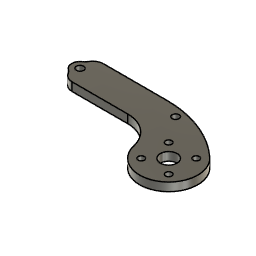
dribbler (Autodesk Fusion 360 archive; units mm, degrees)
design "ドリブラー1-1"
Autodesk Fusion 360 part; units mm, degrees
sketch "スケッチ1" plane through (0, 0, 2.2603) normal (0, 0, -1) x (1, 0, 0)
  circle A0 centre (-0.3584, 25.4794) radius 1.5
  circle A1 centre (12.7938, 12.3272) radius 1.5
  circle A2 centre (6.2177, 18.9033) radius 4
  arc A3 (17.8871, 26.363) -> (13.6774, 30.5727) centre (6.2177, 18.9033) ccw
  arc A4 (-1.242, 30.5727) -> (13.6774, 30.5727) centre (6.2177, 40.3986) ccw
  arc A5 (-1.242, 30.5727) -> (-5.4517, 26.363) centre (6.2177, 18.9033) ccw
  arc A6 (-5.4517, 11.4436) -> (-5.4517, 26.363) centre (-15.2776, 18.9033) ccw
  arc A7 (-5.4517, 11.4436) -> (-1.242, 7.2339) centre (6.2177, 18.9033) ccw
  arc A8 (13.6774, 7.2339) -> (-1.242, 7.2339) centre (6.2177, -2.592) ccw
  arc A9 (13.6774, 7.2339) -> (17.8871, 11.4436) centre (6.2177, 18.9033) ccw
  arc A10 (17.8871, 26.363) -> (17.8871, 11.4436) centre (27.713, 18.9033) ccw
  circle A11 centre (-0.3584, 12.3272) radius 1.5
  circle A12 centre (12.7938, 25.4794) radius 1.5
  circle A13 centre (12.7938, 25.4794) radius 1.6
  circle A14 centre (-0.3584, 12.3272) radius 1.6
  circle A15 centre (12.7938, 12.3272) radius 1.6
  circle A16 centre (-0.3584, 25.4794) radius 1.6
  circle A17 centre (6.2177, 18.9033) radius 13.9
  line L0 (12.7938, 12.3272) -> (-0.3584, 12.3272)
  line L1 (6.2177, 12.3272) -> (6.2177, 10.3272)
  line L2 (6.2177, 10.3272) -> (-53.7823, 10.3272)
  line L3 (6.2177, 18.9033) -> (-0.3584, 12.3272)
  line L4 (-0.3584, 12.3272) -> (-2.3584, 10.3272)
  line L5 (6.2177, 18.9033) -> (-7.6823, 18.9033)
  line L6 (-7.6823, 18.9033) -> (-7.6823, 10.3272)
  line L7 (6.2177, 18.9033) -> (16.0111, 9.1099)
  line L8 (-7.6823, 10.3272) -> (-7.6823, -4.6728)
  line L9 (16.0111, 9.1099) -> (-6.3858, -13.287)
  line L10 (-7.6823, -4.6728) -> (2.2285, -4.6728)
  line L11 (-53.7823, 10.3272) -> (-7.6823, 10.3272)
  line L12 (-7.6823, 10.3272) -> (-7.6823, -4.6728)
  line L13 (-7.6823, -4.6728) -> (-53.7823, -4.6728)
  line L14 (-53.7823, -4.6728) -> (-53.7823, 10.3272)
  dimension "d1" = 3.2
  dimension "d2" = 3.2
  dimension "d3" = 3.2
  dimension "d4" = 3.2
  dimension "d5" = 27.8
  dimension "d8" = 2
  dimension "d9" = 90
  dimension "d10" = 60
  dimension "d11" = 15
  constraint concentric A12 A13
  constraint concentric A11 A14
  constraint concentric A1 A15
  constraint concentric A0 A16
  constraint concentric A2 A17
  constraint coincident A1.centre A15.centre
  constraint coincident A11.centre A14.centre
  constraint midpoint L0 L1.start
  constraint perpendicular L0 L1
  constraint coincident A2.centre A3.centre
  constraint coincident L2 L4.end
  constraint parallel L3 L4
  constraint coincident A17 L5.end
  constraint horizontal L5
  constraint coincident L2 L6.end
  constraint tangent A17 L6
  constraint midpoint A9 L7.end
  constraint perpendicular L2 L8
  constraint tangent A9 L9
  constraint perpendicular L7 L9
  constraint coincident L9 L10.end
  constraint perpendicular L8 L10
  constraint horizontal L11
  constraint vertical L12
  constraint horizontal L13
  constraint vertical L14
  measures "d1" diameter of A13
  measures "d2" diameter of A14
  measures "d3" diameter of A15
  measures "d4" diameter of A16
  measures "d5" diameter of A17
  measures "d8" distance of L1.start L1.end
  measures "d9" angle of L1 L2
  measures "d10" distance of L1.end L2.end
  measures "d11" distance of L6.end L8.end
extrude "押し出し1" add sketch "スケッチ1" along normal blind 4 contours A1 A15 L7 | A1 A15 L0 L7 | A1 A15 L0 L7 | A2 A3 A4 A5 A6 A9 A10 A15 L5 L7 | A2 A14 A15 L0 L3 L7 | A7 A8 A9 A15 L0 L1 L2 L7 | A7 A8 A9 A17 L2 L9 | A3 A4 A5 A6 A9 A10 A17 L5 L9 | A14 L0 L1 L2 L4 | A2 A6 A7 A14 L2 L3 L4 L5 | A17 L2 L8 L9 L10 L12 | A11 A14 L0 L3 | A11 A14 L0 L4 | A11 A14 L3 L4 | A17 L2 L6 | A6 A7 A17 L2 L5 | L2 L8 L11 L12 L13 L14 | A13 | A16
fillet "フィレット1" radius 15 1 edges at (-7.6823, -10.3272, 0.2603)
fillet "フィレット2" radius 50 1 edges at (2.2285, 4.6728, 0.2603)
sketch "スケッチ2" plane through (0, 0, -1.7397) normal (0, 0, -1) x (1, 0, 0)
  arc A0 (-18.3968, -4.6728) -> (15.1782, 8.277) centre (-18.3968, 45.3272) ccw
  arc A1 (15.1782, 8.277) -> (-7.3346, 21.993) centre (6.2177, 18.9033) ccw
  arc A2 (-21.9593, 10.3272) -> (-7.3346, 21.993) centre (-21.9593, 25.3272) ccw
  line L0 (-21.9593, 10.3272) -> (-53.7823, 10.3272)
  line L1 (-53.7823, 10.3272) -> (-53.7823, -4.6728)
  line L2 (-53.7823, -4.6728) -> (-18.3968, -4.6728)
  circle A3 centre (-0.3584, 12.3272) radius 1.5
  circle A4 centre (6.2177, 18.9033) radius 4
  circle A5 centre (12.7938, 25.4794) radius 1.5
  circle A6 centre (-0.3584, 25.4794) radius 1.5
  circle A7 centre (12.7938, 12.3272) radius 1.5
  circle A8 centre (6.2177, 18.9033) radius 13.9
  line L3 (-0.3584, 12.3272) -> (-18.3968, -4.6728)
  line L4 (-9.3776, 3.8272) -> (-9.3776, -3.8526)
  circle A9 centre (-9.3776, -0.0127) radius 3.5
  circle A10 centre (-9.3776, -0.0127) radius 1.65
  dimension "d16" = 7
  dimension "d17" = 3.3
  constraint concentric A1 A8
  constraint coincident A3.centre L3.start
  constraint coincident A0.start L2.end
  constraint midpoint L3 L4.start
  constraint coincident A0 L4.end
  constraint vertical L4
  constraint midpoint L4 A9.centre
  constraint concentric A9 A10
  measures "d16" diameter of A9
  measures "d17" diameter of A10
extrude "押し出し2" cut sketch "スケッチ2" against normal blind 4 contours L4 A10 | L4 A10
extrude "押し出し3" add 1 faces at (-53.7823, -0.3272, 0.927) along direction (-1, 0, 0) blind 6
sketch "スケッチ3" plane through (0, 0, 2.2603) normal (0, 0, 1) x (-1, 0, 0)
  circle A0 centre (9.3776, -0.0127) radius 1.65
  arc A1 (-15.1782, 8.277) -> (18.3968, -4.6728) centre (18.3968, 45.3272) ccw
  line L0 (18.3968, -4.6728) -> (59.7823, -4.6728)
  line L1 (59.7823, -4.6728) -> (59.7823, 10.3272)
  line L2 (59.7823, 10.3272) -> (21.9593, 10.3272)
  arc A2 (7.3346, 21.993) -> (21.9593, 10.3272) centre (21.9593, 25.3272) ccw
  arc A3 (7.3346, 21.993) -> (-15.1782, 8.277) centre (-6.2177, 18.9033) ccw
  circle A4 centre (-12.7938, 12.3272) radius 1.5
  circle A5 centre (0.3584, 25.4794) radius 1.5
  circle A6 centre (-12.7938, 25.4794) radius 1.5
  circle A7 centre (-6.2177, 18.9033) radius 4
  circle A8 centre (0.3584, 12.3272) radius 1.5
  line L3 (59.7823, -4.6728) -> (52.2823, -4.6728)
  line L4 (52.2823, -4.6728) -> (52.2823, 10.3272)
  line L5 (52.2823, 10.3272) -> (59.7823, 10.3272)
  line L6 (59.7823, 10.3272) -> (59.7823, -4.6728)
  circle A9 centre (52.2823, 2.8272) radius 1.75
  circle A10 centre (52.2823, 2.8272) radius 4
  dimension "d22" = 7.5
  dimension "d23" = 15
  dimension "d24" = 3.5
  dimension "d25" = 8
  constraint horizontal L3
  constraint vertical L4
  constraint horizontal L5
  constraint vertical L6
  constraint coincident L0.end L1.start
  constraint midpoint L4 A9.centre
  constraint concentric A9 A10
  measures "d22" distance of L0.end L3.end
  measures "d23" distance of L0.end L1.end
  measures "d24" diameter of A9
  measures "d25" diameter of A10
extrude "押し出し4" cut sketch "スケッチ3" against normal blind 5 contours L0 L1 L2 L3 L4 L5 L6 A10 | L4 A9 | L4 A9
fillet "フィレット3" radius 5 4 edges at (-52.2823, 4.6728, 0.2603) (-52.2823, 1.1728, 0.2603) (-52.2823, -6.8272, 0.2603) (-52.2823, -10.3272, 0.2603)

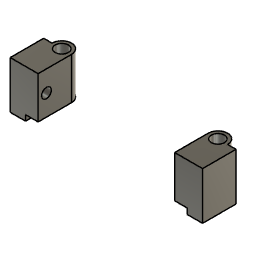
design "ドリブラー1-2"
Autodesk Fusion 360 part; units mm, degrees
sketch "スケッチ1" plane through (0, 0, 0) normal (0, 0, 1) x (1, 0, 0)
  circle A0 centre (0, 0) radius 2.35
  circle A1 centre (0, 0) radius 3.5
  line L0 (0, 0) -> (3.5, 0)
  line L1 (3.5, 0) -> (-6.5, 0)
  line L2 (-6.5, 0) -> (-6.5, -12)
  line L3 (-6.5, -12) -> (3.5, -12)
  line L4 (3.5, -12) -> (3.5, 0)
  dimension "d1" = 4.7
  dimension "d2" = 7
  dimension "d3" = 10
  dimension "d4" = 12
  constraint coincident A0.centre A1.centre
  constraint coincident A1 L0.end
  constraint horizontal L0
  constraint horizontal L1
  constraint vertical L2
  constraint horizontal L3
  constraint vertical L4
  measures "d1" diameter of A0
  measures "d2" diameter of A1
  measures "d3" distance of L0.end L1.end
  measures "d4" distance of L0.end L3.end
  measures "d17" distance of L0.end
extrude "押し出し1" add sketch "スケッチ1" along normal blind 15 contours A0 A1 L0 L1 | A0 A1 L0 L1 | A1 L1 L2 L3 L4 makes body 1
sketch "スケッチ2" plane through (0, 0, 0) normal (0, 0, -1) x (1, 0, 0)
  circle A0 centre (0, 0) radius 2.35
  line L0 (3.5, 0) -> (3.5, 12)
  line L1 (3.5, 12) -> (-6.5, 12)
  line L2 (-6.5, 12) -> (-6.5, 0)
  line L3 (-6.5, 0) -> (-3.5, 0)
  arc A1 (-3.5, 0) -> (3.5, 0) centre (0, 0) ccw
  line L4 (0, 0) -> (-1, 0)
  line L5 (-1, 0) -> (-1, 12)
  line L6 (-6.5, 12) -> (-1, 12)
  line L7 (-1, 12) -> (-1, 0)
  line L8 (-1, 0) -> (-6.5, 0)
  line L9 (-6.5, 0) -> (-6.5, 12)
  circle A2 centre (0, 0) radius 5
  dimension "d7" = 1
  dimension "d10" = 10
  constraint coincident A0.centre A1.centre
  constraint horizontal L4
  constraint coincident L1 L5.end
  constraint perpendicular L1 L5
  constraint horizontal L6
  constraint vertical L7
  constraint horizontal L8
  constraint vertical L9
  constraint coincident L1.end L2.start
  measures "d7" distance of A0.centre L4.end
  measures "d10" diameter of A2
extrude "押し出し2" add sketch "スケッチ2" along normal blind 2 contours L1 L2 L3 L5 L6 L7 L8 L9 A2 bodies 1
sketch "スケッチ3" plane through (-6.5, 0, 0) normal (-1, 0, 0) x (0, -1, 0)
  line L0 (12, -2) -> (12, 15)
  line L1 (12, 15) -> (0, 15)
  line L2 (0, 15) -> (0, -2)
  line L3 (0, -2) -> (12, -2)
  line L4 (0, 0) -> (12.3256, 0)
  line L5 (0, 0) -> (12, 15)
  line L6 (0, 15) -> (12, 0)
  line L7 (6, 7.5) -> (12, 7.5)
  circle A0 centre (9, 7.5) radius 1.75
  dimension "d11" = 3.5
  constraint coincident L4.start L5.start
  constraint perpendicular L0 L4
  constraint coincident L0.end L1.start
  constraint coincident L1.end L2.start
  constraint coincident L4 L6.end
  constraint coincident L0 L6.end
  constraint midpoint L5 L7.start
  constraint coincident L0 L7.end
  constraint perpendicular L0 L7
  constraint midpoint L7 A0.centre
  measures "d11" diameter of A0
extrude "押し出し3" cut sketch "スケッチ3" against normal blind 13 contours L7 A0 | L7 A0 bodies 1
copy_body "ボディのコピーと貼り付け1" bodies 1 makes body 2
move_body "移動1" bodies 2 to x (1, 0, 0) y (0, 1, 0) z (0, 0, 1) at (50, 0, 0)
sketch "スケッチ4" plane through (0, 0, 15) normal (0, 0, 1) x (-1, 0, 0)
  circle A0 centre (-50, 0) radius 2.35
  line L0 (-53.5, 12) -> (-53.5, 0)
  arc A1 (-53.5, 0) -> (-46.5, 0) centre (-50, 0) ccw
  line L1 (-46.5, 0) -> (-43.5, 0)
  line L2 (-43.5, 0) -> (-43.5, 12)
  line L3 (-43.5, 12) -> (-53.5, 12)
  line L4 (-46.5, 0) -> (-43.5, 0)
  line L5 (-43.5, 0) -> (-43.5, 12)
  line L6 (-43.5, 12) -> (-46.5, 12)
  line L7 (-46.5, 12) -> (-46.5, 0)
  line L8 (-53.5, 0) -> (-56.5, 0)
  line L9 (-56.5, 0) -> (-56.5, 12)
  line L10 (-56.5, 12) -> (-53.5, 12)
  line L11 (-53.5, 12) -> (-53.5, 0)
  dimension "d14" = 3
  constraint horizontal L4
  constraint vertical L5
  constraint horizontal L6
  constraint vertical L7
  constraint coincident L2.end L3.start
  constraint coincident A1.end L1.start
  constraint horizontal L8
  constraint vertical L9
  constraint horizontal L10
  constraint vertical L11
  constraint coincident L0.end A1.start
  measures "d14" distance of L0.end L8.end
extrude "押し出し4" add sketch "スケッチ4" against normal blind 15 contours L0 L8 L9 L10 L11 bodies 2
sketch "スケッチ5" plane through (0, 0, 0) normal (0, 0, -1) x (1, 0, 0)
  arc A0 (49, 4.899) -> (45, 0) centre (50, 0) ccw
  line L0 (45, 0) -> (46.5, 0)
  arc A1 (46.5, 0) -> (53.5, 0) centre (50, 0) ccw
  line L1 (53.5, 0) -> (56.5, 0)
  line L2 (56.5, 0) -> (56.5, 12)
  line L3 (56.5, 12) -> (49, 12)
  line L4 (49, 12) -> (49, 4.899)
  circle A2 centre (50, 0) radius 2.35
  circle A3 centre (50, 0) radius 5
  line L5 (50, 0) -> (50, 5)
  line L6 (50, 5) -> (51, 5)
  line L7 (56.5, 12) -> (51, 12)
  line L8 (51, 12) -> (51, 5)
  line L9 (51, 5) -> (56.5, 5)
  line L10 (56.5, 5) -> (56.5, 12)
  line L11 (51, 5) -> (56.5, 5)
  line L12 (56.5, 5) -> (56.5, 0)
  line L13 (56.5, 0) -> (51, 0)
  line L14 (51, 0) -> (51, 5)
  dimension "d17" = 1
  constraint concentric A0 A3
  constraint coincident A0.start A3
  constraint coincident A0.centre A1.centre
  constraint coincident A3 L5.end
  constraint vertical L5
  constraint perpendicular L4 L6
  constraint horizontal L7
  constraint vertical L8
  constraint horizontal L9
  constraint vertical L10
  constraint coincident L2.end L3.start
  constraint horizontal L11
  constraint vertical L12
  constraint horizontal L13
  constraint vertical L14
  constraint coincident L1.end L2.start
  measures "d17" distance of L5.end L6.end
extrude "押し出し5" add sketch "スケッチ5" along normal blind 2 contours L1 L2 A3 L9 L11 L12 L13 L14 | L2 L3 L7 L8 L9 L10 L11 bodies 2
sketch "スケッチ6" plane through (0, 0, 15) normal (0, 0, 1) x (-1, 0, 0)
  circle A0 centre (-50, 0) radius 2.35
  arc A1 (-53.5, 0) -> (-46.5, 0) centre (-50, 0) ccw
  line L0 (-46.5, 0) -> (-43.5, 0)
  line L1 (-43.5, 0) -> (-43.5, 12)
  line L2 (-43.5, 12) -> (-56.5, 12)
  line L3 (-56.5, 12) -> (-56.5, 0)
  line L4 (-56.5, 0) -> (-53.5, 0)
  line L5 (-46.5, 0) -> (-43.5, 0)
  line L6 (-43.5, 0) -> (-43.5, 12)
  line L7 (-43.5, 12) -> (-46.5, 12)
  line L8 (-46.5, 12) -> (-46.5, 0)
  constraint horizontal L5
  constraint vertical L6
  constraint horizontal L7
  constraint vertical L8
  constraint coincident L1.end L2.start
  constraint coincident A1.end L0.start
extrude "押し出し6" cut sketch "スケッチ6" against normal blind 21 contours L0 L1 L2 L5 L6 L7 L8 bodies 2
extrude "押し出し7" cut 1 faces at (48.1667, -9.633, -2) along direction (0, 0, 1) blind 2 on bodies 2 bodies 2
move_body "移動2" bodies 2 to x (1, 0, 0) y (0, 1, 0) z (0, 0, 1) at (6, 0, 0)
